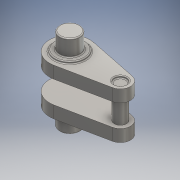
# Autodesk Inventor part: Crank
Saved by Autodesk Inventor 2016 (Build 200138000, 138)
## iProperties
Created: 2017-07-15
Part Number: Crank
Material: Steel, Carbon
Document SubType Name: Modeling
Designer: bobbyl
Density: 7.85 g/cm^3
Appearance: Semi-Polished
Mass: 553.342 g
Surface Area: 167.793 cm^2
Volume: 70.4895 cm^3
Author: bobbyl
Autodesk Inventor part; units mm, degrees
ref_plane "YZ Plane" through (0, 0, 0) normal (1, 0, 0) x (0, 1, 0)
ref_plane "XZ Plane" through (0, 0, 0) normal (0, 1, 0) x (-1, 0, 0)
sketch "Sketch1" plane through (0, 0, 0) normal (0, 0, 1) x (1, 0, 0)
  circle A0 centre (0, 0) radius 6
  dimension "d0" = 12
  constraints: 1 centre point, 1 coincident
  measures "d0" diameter of A0
extrude "Extrusion1" add sketch "Sketch1" along normal blind 21
ref_plane "Work Plane1" through (0, 0, 11) normal (0, 0, 1) x (1, 0, 0)
sketch "Sketch2" plane through (0, 0, 11) normal (0, 0, 1) x (1, 0, 0)
  arc A0 (2, -9.798) -> (2, 9.798) centre (0, 0) ccw
  arc A1 (-46, 19.5959) -> (-46, -19.5959) centre (-50, 0) ccw
  line L0 (-86, 0) -> (26, 0) projected
  line L1 (2, 9.798) -> (-46, 19.5959)
  line L2 (2, -9.798) -> (-46, -19.5959)
  circle A2 centre (0, 0) radius 6 projected
  circle A3 centre (0, 0) radius 6
  dimension "d4" = 20
  dimension "d5" = 40
  dimension "d6" = 50
  constraints: 4 end point, 4 point on circle, 4 tangent, 3 centre point, 2 coincident, 1 concentric, 1 point on line
  measures "d4" diameter of A0
  measures "d5" diameter of A1
  measures "d6" distance of A1.centre point (0, 0)
extrude "Extrusion2" add sketch "Sketch2" along normal blind 12 contours L2 A1 L0 A2 A0 | L0 A2 A1 L1 A0
sketch "Sketch3" plane through (0, 0, 23) normal (0, 0, 1) x (1, 0, 0)
  circle A0 centre (-50, 0) radius 15
  circle A1 centre (0, 0) radius 6 projected
  arc A2 (2, -9.798) -> (2, 9.798) centre (0, 0) ccw projected
  line L0 (2, 9.798) -> (-46, 19.5959) projected
  arc A3 (-46, 19.5959) -> (-46, -19.5959) centre (-50, 0) ccw projected
  line L1 (-46, -19.5959) -> (2, -9.798) projected
  dimension "d9" = 30
  constraints: 1 centre point, 1 concentric
  measures "d9" diameter of A0
extrude "Extrusion3" add sketch "Sketch3" along normal blind 2 contours A0
sketch "Sketch4" plane through (-50, 0, 25) normal (0, 0, 1) x (1, 0, 0)
  circle A0 centre (0, 0) radius 10
  circle A1 centre (0, 0) radius 15 projected
  point P0 (50, 0)
  dimension "d12" = 20
  constraints: 1 centre point, 1 concentric
  measures "d12" diameter of A0
extrude "Extrusion4" add sketch "Sketch4" along normal blind 16 contours A0
fillet "Fillet1" radius 1 6 edges at (-6, 0, 23) (-65, 0, 25) (-60, 0, 41) (-6, 0, 21) (-65, 0, 23) (-60, 0, 25)
mirror "Mirror1" about plane through (0, 0, 0) normal (0, 0, 1) of "Extrusion1", "Extrusion2", "Extrusion3", "Extrusion4", "Fillet1"
body "Solid1"
